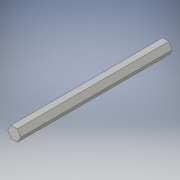
# Autodesk Inventor part: Hex Shaft 2
Saved by Autodesk Inventor 2016 (Build 200138000, 138)
## iProperties
Created: 2016-03-19
Part Number: Hex Shaft 2
Material: Generic
Document SubType Name: Modeling
Designer: matth_000
Density: 1 g/cm^3
Appearance: Default
Author: matth_000
Autodesk Inventor part; units mm, degrees
ref_plane "YZ Plane" through (0, 0, 0) normal (1, 0, 0) x (0, 1, 0)
ref_plane "XZ Plane" through (0, 0, 0) normal (0, 1, 0) x (-1, 0, 0)
ref_plane "XY Plane" through (0, 0, 0) normal (0, 0, 1) x (1, 0, 0)
sketch "Sketch1" plane through (0, 0, 0) normal (0, 0, 1) x (1, 0, 0)
  line L0 (-7.3288, -0.2277) -> (-3.8616, 6.2331)
  line L1 (-3.8616, 6.2331) -> (3.4672, 6.4608)
  line L2 (3.4672, 6.4608) -> (7.3288, 0.2277)
  line L3 (7.3288, 0.2277) -> (3.8616, -6.2331)
  line L4 (3.8616, -6.2331) -> (-3.4672, -6.4608)
  line L5 (-3.4672, -6.4608) -> (-7.3288, -0.2277)
  point P0 (0, 0)
  point P1 (0, 0)
  dimension "d0" = 12.7
  constraints: 12 end point, 1 coincident, 13 other
  measures "d0" distance between parallel lines of L4 L1
extrude "Extrusion1" add sketch "Sketch1" along normal blind 169.545
body "Solid1"
